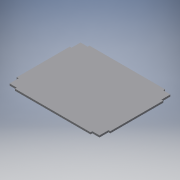
# Autodesk Inventor part: top
Saved by Autodesk Inventor 2018 (Build 220112000, 112)
## iProperties
Created: 2017-10-09
Part Number: top
Material: Generic
Document SubType Name: Modeling
Designer: HP
Density: 1 g/cm^3
Appearance: Fine Textured - Black
Author: HP
Autodesk Inventor part; units mm, degrees
ref_plane "YZ Plane" through (0, 0, 0) normal (1, 0, 0) x (0, 1, 0)
ref_plane "XZ Plane" through (0, 0, 0) normal (0, 1, 0) x (-1, 0, 0)
ref_plane "XY Plane" through (0, 0, 0) normal (0, 0, 1) x (1, 0, 0)
sketch "Sketch1" plane through (0, 0, 0) normal (0, 0, 1) x (1, 0, 0)
  line L0 (-236.1, 0) -> (-211.2, 0) construction
  line L1 (-211.2, 0) -> (-211.2, 5) construction
  line L2 (-236.1, 5) -> (-211.2, 5) construction
  line L3 (-236.1, 0) -> (-236.1, 5) construction
  circle A0 centre (-20, 2.5) radius 1.2295 construction
  circle A1 centre (-105.6, 2.5) radius 1.2295 construction
  circle A2 centre (-191.2, 2.5) radius 1.2295 construction
  line L4 (-211.2, 0) -> (0, 0) construction
  line L5 (0, 0) -> (0, 5) construction
  line L6 (-211.2, 5) -> (0, 5) construction
  line L7 (-211.2, 0) -> (-211.2, 5) construction
  line L8 (0, 0) -> (24.9, 0) construction
  line L9 (24.9, 0) -> (24.9, 5) construction
  line L10 (0, 5) -> (24.9, 5) construction
  line L11 (0, 0) -> (0, 5) construction
  line L12 (19.9, -0.1) -> (19.9, -25) construction
  line L13 (19.9, -25) -> (24.9, -25) construction
  line L14 (24.9, -0.1) -> (24.9, -25) construction
  line L15 (19.9, -0.1) -> (24.9, -0.1) construction
  circle A3 centre (22.4, -45) radius 1.2295 construction
  circle A4 centre (22.4, -99) radius 1.2295 construction
  circle A5 centre (22.4, -153) radius 1.2295 construction
  line L16 (19.9, -25) -> (19.9, -173) construction
  line L17 (19.9, -173) -> (24.9, -173) construction
  line L18 (24.9, -25) -> (24.9, -173) construction
  line L19 (19.9, -25) -> (24.9, -25) construction
  line L20 (-236.1, -0.1) -> (-236.1, -25) construction
  line L21 (-236.1, -25) -> (-231.1, -25) construction
  line L22 (-231.1, -0.1) -> (-231.1, -25) construction
  line L23 (-236.1, -0.1) -> (-231.1, -0.1) construction
  circle A6 centre (-233.6, -45) radius 1.2295 construction
  circle A7 centre (-233.6, -99) radius 1.2295 construction
  circle A8 centre (-233.6, -153) radius 1.2295 construction
  line L24 (-236.1, -25) -> (-236.1, -173) construction
  line L25 (-236.1, -173) -> (-231.1, -173) construction
  line L26 (-231.1, -25) -> (-231.1, -173) construction
  line L27 (-236.1, -25) -> (-231.1, -25) construction
  line L28 (-236.1, -173) -> (-236.1, -197.9) construction
  line L29 (-236.1, -197.9) -> (-231.1, -197.9) construction
  line L30 (-231.1, -173) -> (-231.1, -197.9) construction
  line L31 (-236.1, -173) -> (-231.1, -173) construction
  line L32 (-211.2, -198) -> (-236.1, -198) construction
  line L33 (-236.1, -198) -> (-236.1, -203) construction
  line L34 (-211.2, -203) -> (-236.1, -203) construction
  line L35 (-211.2, -198) -> (-211.2, -203) construction
  circle A9 centre (-191.2, -200.5) radius 1.2295 construction
  circle A10 centre (-105.6, -200.5) radius 1.2295 construction
  circle A11 centre (-20, -200.5) radius 1.2295 construction
  line L36 (0, -198) -> (-211.2, -198) construction
  line L37 (-211.2, -198) -> (-211.2, -203) construction
  line L38 (0, -203) -> (-211.2, -203) construction
  line L39 (0, -198) -> (0, -203) construction
  line L40 (24.9, -198) -> (0, -198) construction
  line L41 (0, -198) -> (0, -203) construction
  line L42 (24.9, -203) -> (0, -203) construction
  line L43 (24.9, -198) -> (24.9, -203) construction
  line L44 (19.9, -173) -> (19.9, -197.9) construction
  line L45 (19.9, -197.9) -> (24.9, -197.9) construction
  line L46 (24.9, -173) -> (24.9, -197.9) construction
  line L47 (19.9, -173) -> (24.9, -173) construction
  line L48 (-0.1, -203) -> (-211.1, -203)
  line L49 (-211.1, -198) -> (-231.1, -198)
  line L50 (-231.1, -198) -> (-231.1, -172.9)
  line L51 (-236.1, -172.9) -> (-236.1, -25.1)
  line L52 (-231.1, -25) -> (-231.1, 0)
  line L53 (-231.1, 0) -> (-211.2, 0)
  line L54 (-211.1, 5) -> (-0.1, 5)
  line L55 (0, 0) -> (19.9, 0)
  line L56 (19.9, 0) -> (19.9, -25)
  line L57 (24.9, -25.1) -> (24.9, -172.9)
  line L58 (19.9, -173) -> (19.9, -198)
  line L59 (19.9, -198) -> (-0.1, -198)
  line L60 (-236.1, -172.9) -> (-231.1, -172.9)
  line L61 (-211.1, -198) -> (-211.1, -203)
  line L62 (-0.1, -203) -> (-0.1, -198)
  line L63 (19.9, -172.9) -> (24.9, -172.9)
  line L64 (19.9, -173) -> (19.9, -172.9)
  line L65 (19.9, -25.1) -> (24.9, -25.1)
  line L66 (19.9, -25) -> (19.9, -25.1)
  line L67 (-0.1, 5) -> (-0.1, 0)
  line L68 (-0.1, 0) -> (0, 0)
  line L69 (-211.1, 5) -> (-211.1, 0)
  line L70 (-211.1, 0) -> (-211.2, 0)
  line L71 (-236.1, -25.1) -> (-231.1, -25.1)
  line L72 (-231.1, -25) -> (-231.1, -25.1)
  dimension "d0" = 0.1
  dimension "d1" = 0.1
  dimension "d2" = 0.1
  dimension "d3" = 0.1
  dimension "d4" = 0.1
  dimension "d5" = 0.1
  dimension "d6" = 0.1
  dimension "d7" = 0.1
  constraints: 50 end point, 14 collinear, 14 point on line, 9 perpendicular, 1 horizontal
  measures "d0" distance between parallel lines of L25 L60
  measures "d1" distance between parallel lines of L35 L61
  measures "d2" distance between parallel lines of L41 L62
  measures "d3" distance between parallel lines of L17 L63
  measures "d4" distance between parallel lines of L13 L65
  measures "d5" distance between parallel lines of L5 L67
  measures "d6" distance between parallel lines of L1 L69
  measures "d7" distance between parallel lines of L21 L71
extrude "Extrusion1" add sketch "Sketch1" against normal blind 5
sketch "Sketch2" plane through (0, 0, 0) normal (0, 0, 1) x (1, 0, 0)
  circle A0 centre (-20, -200.5) radius 1.2295 construction
  circle A1 centre (-105.6, -200.5) radius 1.2295 construction
  circle A2 centre (-191.2, -200.5) radius 1.2295 construction
  circle A3 centre (-233.6, -153) radius 1.2295 construction
  circle A4 centre (-233.6, -99) radius 1.2295 construction
  circle A5 centre (-233.6, -45) radius 1.2295 construction
  circle A6 centre (-191.2, 2.5) radius 1.2295 construction
  circle A7 centre (-105.6, 2.5) radius 1.2295 construction
  circle A8 centre (-20, 2.5) radius 1.2295 construction
  circle A9 centre (22.4, -45) radius 1.2295 construction
  circle A10 centre (22.4, -99) radius 1.2295 construction
  circle A11 centre (22.4, -153) radius 1.2295 construction
  point P0 (0, 0)
hole "Hole1" at (-233.6, -153, 0) at (-233.6, -99, 0) at (-233.6, -45, 0) at (-191.2, 2.5, 0) at (-191.2, -200.5, 0) at (-105.6, -200.5, 0) at (-20, -200.5, 0) at (22.4, -153, 0) at (22.4, -99, 0) at (22.4, -45, 0) at (-105.6, 2.5, 0) at (-20, 2.5, 0) direction (0, 0, -1) diameter 3 end through all
sketch "Sketch3" plane through (0, 0, 0) normal (0, 0, 1) x (1, 0, 0)
  line L0 (-225.6, -127.5) -> (-225.6, -167.5) construction
  line L1 (-225.6, -167.5) -> (-133.7686, -186.657) construction
  arc A0 (-133.7686, -186.657) -> (-133.7686, -108.343) centre (-125.6, -147.5) ccw construction
  line L2 (-133.7686, -108.343) -> (-225.6, -127.5) construction
  line L3 (-134.177, -188.6149) -> (-227.6, -169.1258)
  line L4 (-227.6, -169.1258) -> (-227.6, -125.8742)
  line L5 (-227.6, -125.8742) -> (-134.177, -106.3851)
  arc A1 (-134.177, -188.6149) -> (-134.177, -106.3851) centre (-125.6, -147.5) ccw
  circle A2 centre (-202.6, -97.5) radius 12.5
  point P0 (0, 0)
  dimension "d17" = 2
  dimension "d18" = 50
  dimension "d19" = 25
  dimension "d20" = 25
  constraints: 6 end point, 2 centre point, 2 point on circle, 3 other
  measures "d17" distance between parallel lines of L1 L3
  measures "d18" vertical distance of A0.centre A2.centre
  measures "d19" distance from line of A2.centre L4
  measures "d20" diameter of A2
extrude "Extrusion2" cut sketch "Sketch3" against normal through all
equation "\"d0\" = ABS_tolerance"
equation "\"d1\" = ABS_tolerance"
equation "\"d2\" = ABS_tolerance"
equation "\"d3\" = ABS_tolerance"
equation "\"d4\" = ABS_tolerance"
equation "\"d5\" = ABS_tolerance"
equation "\"d6\" = ABS_tolerance"
equation "\"d7\" = ABS_tolerance"
equation "\"d8\" = plate_thickness"
equation "\"plate_thickness\" = 5"
equation "\"basic_plate_offset\" = 0.5"
equation "\"ABS_tolerance\" = 0.1"
equation "\"laser_cutter_thickness\" = 0.1"
body "Solid1"
